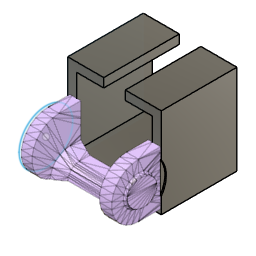
bed_end_chain (Autodesk Fusion 360 design; units mm, degrees)
Autodesk Fusion 360 part; units mm, degrees
sketch "Sketch1" plane through (0, 0, 0) normal (0, 0, 1) x (1, 0, 0)
  line L0 (8.4, 8.4) -> (-8.4, 8.4)
  line L1 (-8.4, 8.4) -> (-8.4, -8.4)
  line L2 (-8.4, -8.4) -> (8.4, -8.4)
  line L3 (8.4, -8.4) -> (8.4, 8.4)
  line L4 (8.4, 8.4) -> (-8.4, -8.4) construction
  line L5 (-8.4, 8.4) -> (8.4, -8.4) construction
  line L6 (8.4, -8.4) -> (10.4, -8.4)
  line L7 (10.4, -8.4) -> (10.4, 8.4)
  line L8 (8.4, 6.6) -> (8.4, -8.4)
  line L9 (-8.4, -8.4) -> (-10.4, -8.4)
  line L10 (-10.4, -8.4) -> (-10.4, 8.4)
  line L11 (-8.4, 6.6) -> (-8.4, -8.4)
  line L12 (-8.4, 8.4) -> (-8.4, 6.6)
  line L13 (8.4, 8.4) -> (8.4, 6.6)
  line L14 (-10.4, 8.4) -> (-8.4, 8.4)
  line L15 (8.4, 8.4) -> (10.4, 8.4)
  dimension "d1" = 16.8
  dimension "d2" = 16.8
  dimension "d3" = 2
  dimension "d4" = 15
  dimension "d5" = 2
  dimension "d6" = 15
  dimension "d21" = 16.8
  dimension "d22" = 16.8
  constraint horizontal L0
  constraint perpendicular L0 L1
  constraint parallel L0 L2
  constraint parallel L1 L3
  constraint coincident L4 origin
  constraint coincident L5 origin
  constraint horizontal L6
  constraint vertical L7
  constraint vertical L8
  constraint horizontal L9
  constraint vertical L10
  constraint vertical L11
  constraint vertical L12
  constraint vertical L13
  measures "d1" distance of L1.end L2.end
  measures "d2" distance of L0.end L1.end
  measures "d3" distance of L2.end L6.end
  measures "d4" distance of L2.end L8.start
  measures "d5" distance of L1.end L9.end
  measures "d6" distance of L1.end L11.start
  measures "d21" distance of L9.end L10.end
  measures "d22" distance of L6.end L7.end
extrude "Extrude1" add sketch "Sketch1" along normal blind 3 contours L0 L1 L2 L3 L8 L11 L12 L13
extrude "Extrude2" add sketch "Sketch1" along normal blind 18 contours L3 L6 L7 L8 L13 L15 | L1 L9 L10 L11 L12 L14
other "Base Mesh Feature1"
other "MeshPlaneCut1"
other "Modify1"
other "Modify2"
other "Modify3"
sketch "Sketch2" plane through (0, -8.4, 0) normal (0, -1, 0) x (1, 0, 0)
  line L0 (-10.4, 0) -> (10.4, 0)
  line L1 (10.4, 0) -> (10.4, 18)
  line L2 (10.4, 18) -> (8.4, 18)
  line L3 (8.4, 18) -> (8.4, 3)
  line L4 (8.4, 3) -> (-8.4, 3)
  line L5 (-8.4, 3) -> (-8.4, 18)
  line L6 (-8.4, 18) -> (-10.4, 18)
  line L7 (-10.4, 18) -> (-10.4, 0)
  line L8 (-10.4, 18) -> (-2.4, 18)
  line L9 (-2.4, 18) -> (-2.4, 20)
  line L10 (-2.4, 20) -> (-10.4, 20)
  line L11 (-10.4, 20) -> (-10.4, 18)
  line L12 (10.4, 18) -> (2.4, 18)
  line L13 (2.4, 18) -> (2.4, 20)
  line L14 (2.4, 20) -> (10.4, 20)
  line L15 (10.4, 20) -> (10.4, 18)
  dimension "d15" = 8
  dimension "d16" = 2
  dimension "d17" = 8
  dimension "d18" = 2
  constraint horizontal L8
  constraint vertical L9
  constraint horizontal L10
  constraint vertical L11
  constraint coincident L6.end L7.start
  constraint horizontal L12
  constraint vertical L13
  constraint horizontal L14
  constraint vertical L15
  constraint coincident L1.end L2.start
  measures "d15" distance of L6.end L8.end
  measures "d16" distance of L6.end L10.end
  measures "d17" distance of L1.end L12.end
  measures "d18" distance of L1.end L14.end
extrude "Extrude3" add sketch "Sketch2" against normal blind 16.8 contours L6 L8 L9 L10 L11 | L2 L12 L13 L14 L15
other "MeshPlaneCut2"
other "MeshPlaneCut3"
other "Base Mesh Feature3"
other "MeshPlaneCut4"
other "Modify4"
other "Modify5"
sketch "Sketch3" plane through (-10.4, 0, 0) normal (-1, 0, 0) x (0, -1, 0)
  line L0 (-8.4, 0) -> (8.4, 0)
  line L1 (8.4, 0) -> (8.4, 20)
  line L2 (8.4, 20) -> (-8.4, 20)
  line L3 (-8.4, 20) -> (-8.4, 0)
  circle A0 centre (13.2443, 7.025) radius 5.9554
extrude "Extrude4" cut sketch "Sketch3" against normal blind 0.5 contours L1 A0 picked at (8.2566, 7.9466)
extrude "Extrude5" cut sketch "Sketch3" along normal blind -20.5 and the other way blind 23 contours L1 A0 picked at (8.2566, 7.9466)
